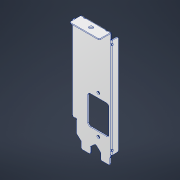
# Autodesk Inventor part: power_ac_plate
Saved by Autodesk Inventor 2022 (Build 260153000, 153)
## iProperties
Created: 2025-03-03
Part Number: power_ac_plate
Material: アルミニウム 6061
Document SubType Name: Sheet Metal
Designer: gisen
Density: 2.7 g/cm^3
Sheet Metal Rule: Default_mm
Appearance: アルミニウム - フラット
Author: gisen
Autodesk Inventor part; units mm, degrees
ref_plane "YZ Plane" through (0, 0, 0) normal (1, 0, 0) x (0, 1, 0)
ref_plane "XZ Plane" through (0, 0, 0) normal (0, 1, 0) x (-1, 0, 0)
ref_plane "XY Plane" through (0, 0, 0) normal (0, 0, 1) x (1, 0, 0)
sketch "スケッチ1" plane through (0, 0, 0) normal (0, 0, 1) x (1, 0, 0)
  line L0 (0, 11.925) -> (5.45, 7)
  line L1 (5.45, 7) -> (5.45, 0)
  line L2 (5.45, 0) -> (14.95, 0)
  line L3 (14.95, 0) -> (14.95, 7)
  line L4 (14.95, 7) -> (17, 8.8525)
  line L5 (17, 8.8525) -> (17, 119.9)
  line L6 (17, 119.9) -> (0, 119.9)
  line L7 (0, 119.9) -> (0, 11.925) construction
  line L8 (0, 11.925) -> (-5.45, 7)
  line L9 (-5.45, 7) -> (-5.45, 0)
  line L10 (-5.45, 0) -> (-14.95, 0)
  line L11 (-14.95, 0) -> (-14.95, 7)
  line L12 (-14.95, 7) -> (-17, 8.8525)
  line L13 (-17, 8.8525) -> (-17, 119.9)
  line L14 (-17, 119.9) -> (0, 119.9)
  point P0 (0, 0)
  dimension "d0" = 9.5
  dimension "d2" = 11.925
  dimension "d3" = 7
  dimension "d4" = 119.9
  dimension "d73" = 132.103
  dimension "d74" = 132.103
  dimension "d75" = 34
  measures "d0" distance of L1.end L2.end
  measures "d2" distance from line of L2 L0.start
  measures "d3" distance of L0.end L1.end
  measures "d4" distance between parallel lines of L2 L6
  measures "d73" angle of L1 L0
  measures "d74" angle of L3 L4
  measures "d75" distance between parallel lines of L5 L13
extrude "プレート1" add sketch "スケッチ1" along normal blind 1
sketch "スケッチ3" plane through (0, 0, 1) normal (0, 0, 1) x (1, 0, 0)
  line L0 (-17, 119.9) -> (17, 119.9) construction
  line L1 (-17, 8.8525) -> (-17, 119.9) construction
  line L2 (17, 119.9) -> (17, 8.8525) construction
  line L3 (0, 11.925) -> (0, 119.9) construction
  line L4 (-17, 64.3763) -> (17, 64.3763) construction
  line L5 (-8.05, 55.125) -> (14.05, 55.125)
  line L6 (14.05, 55.125) -> (14.05, 24.725)
  line L7 (14.05, 24.725) -> (-8.05, 24.725)
  line L8 (-8.05, 24.725) -> (-8.05, 55.125)
  line L9 (3, 59.925) -> (3, 19.925) construction
  circle A0 centre (3, 59.925) radius 1.55
  circle A1 centre (3, 19.925) radius 1.55
  point P0 (0, 0)
  point P1 (-8.05, 39.925)
  point P2 (3, 39.925)
  point P3 (3, 55.125)
  dimension "d77" = 22.1
  dimension "d78" = 30.4
  dimension "d79" = 40
  dimension "d80" = 3.1
  dimension "d83" = 3
  dimension "d84" = 8
  constraints: 14 end point, 6 midpoint, 2 centre point, 2 coincident, 2 parallel, 1 equal radius, 1 horizontal, 1 horizontal alignment, 1 perpendicular, 1 point on line, 1 vertical
  measures "d77" distance of L6.end L7.end
  measures "d78" distance of L5.end L6.end
  measures "d79" distance of L9.start L9.end
  measures "d80" diameter of A0
  measures "d83" distance between parallel lines of L9 L3
  measures "d84" vertical distance of L9.end L3.start
extrude "切り取り1" cut sketch "スケッチ3" against normal blind 1
sketch "スケッチ4" plane through (0, 0, 1) normal (0, 0, 1) x (1, 0, 0)
  line L0 (17, 119.9) -> (15.5, 119.9)
  line L1 (15.5, 119.9) -> (15.5, 114.3)
  line L2 (15.5, 114.3) -> (17, 114.3)
  line L3 (17, 114.3) -> (17, 119.9)
  line L4 (14.95, 7) -> (14.95, 0) construction
  line L5 (-17, 119.9) -> (-15.5, 119.9)
  line L6 (-15.5, 119.9) -> (-15.5, 114.3)
  line L7 (-15.5, 114.3) -> (-17, 114.3)
  line L8 (-17, 114.3) -> (-17, 119.9)
  point P0 (0, 0)
  dimension "d14" = 5.6
  dimension "d76" = 1.5
  constraints: 16 end point, 4 parallel, 2 equal length, 2 horizontal, 2 perpendicular
  measures "d14" distance of L0.end L1.end
  measures "d76" distance of L1.end L2.end
extrude "切り取り2" cut sketch "スケッチ4" against normal blind 1
sketch "スケッチ5" plane through (0, 0, 1) normal (0, 0, 1) x (1, 0, 0)
  line L0 (17, 8.8525) -> (14.95, 7) construction
  line L1 (17, 114.3) -> (17, 8.8525) construction
  line L2 (15.5, 7.497) -> (15.5, 10)
  line L3 (15.5, 10) -> (17, 10)
  line L4 (15.5, 7.497) -> (17, 8.8525)
  line L5 (17, 8.8525) -> (17, 10)
  line L6 (14.95, 7) -> (14.95, 0) projected
  line L7 (14.95, 0) -> (5.45, 0) projected
  line L8 (0, 11.925) -> (0, 120.3299) construction
  line L9 (-17, 8.8525) -> (-14.95, 7) construction
  line L10 (-15.5, 7.497) -> (-15.5, 10)
  line L11 (-15.5, 10) -> (-17, 10)
  line L12 (-15.5, 7.497) -> (-17, 8.8525)
  line L13 (-17, 8.8525) -> (-17, 10)
  line L14 (15.5, 114.3) -> (15.5, 119.9) construction
  point P0 (0, 0)
  dimension "d18" = 10
  constraints: 20 end point, 5 symmetric about line, 4 point on line, 2 vertical, 1 perpendicular
  measures "d18" distance between parallel lines of L7 L3
extrude "切り取り3" cut sketch "スケッチ5" against normal blind 1 contours L2 L3 L5 L4
sketch "スケッチ7" plane through (-15.5, 119.901, 1.001) normal (0, 1, 0) x (-1, 0, 0)
  line L0 (-31, 0) -> (0, 0)
  line L1 (0, 0) -> (0, 11.599)
  line L2 (0, 11.599) -> (-31, 11.599)
  line L3 (-31, 11.599) -> (-31, 0)
  constraints: 6 end point, 1 horizontal, 1 perpendicular, 1 vertical
edge flange "フランジ1" height 11.6 angle 90 thickness 1 bend radius 0 thickness toward (0, 1, 0) relief straight relief width 1 relief depth 0.5 edges at (0, 119.9, 1) wall of the first edge with corners at (15.5, 119.901, 1.001) (-15.5, 119.901, 1.001) (-15.5, 119.901, 12.6) (15.5, 119.901, 12.6)
bend "曲げ2"
corner "コーナー1"
sketch "スケッチ8" plane through (16, 10, 1) normal (1, 0, 0) x (0, 1, 0)
  line L0 (104.3, 0) -> (0, 0)
  line L1 (0, 0) -> (0, -7)
  line L2 (0, -7) -> (104.3, -7)
  line L3 (104.3, -7) -> (104.3, 0)
  constraints: 6 end point, 1 horizontal, 1 perpendicular, 1 vertical
edge flange "フランジ2" height 6 angle 90 thickness 1 bend radius 0 thickness toward (1, 0, 0) relief straight relief width 1 relief depth 0.5 edges at (17, 62.15, 0) wall of the first edge with corners at (16, 114.3, 1) (16, 10, 1) (16, 10, -6) (16, 114.3, -6)
bend "曲げ3"
corner "コーナー2"
sketch "スケッチ15" plane through (0, 0, 1) normal (0, 0, 1) x (1, 0, 0)
  line L0 (-17, 8.8525) -> (-17, 114.3)
  line L1 (-14.95, 7) -> (-17, 8.8525) construction
  line L2 (-17, 8.8525) -> (-24, 15.1782)
  line L3 (-24, 15.1782) -> (-24, 114.3)
  line L4 (-24, 114.3) -> (-17, 114.3)
  line L5 (-24, 25) -> (-20, 25)
  line L6 (-20, 25) -> (-20, 11.5635)
  line L7 (-5.45, 0) -> (-14.95, 0)
  point P0 (0, 0)
  dimension "d98" = 7
  dimension "d105" = 4
  dimension "d106" = 25
  measures "d98" distance of L3.end L0.end
  measures "d105" distance of L5.start L5.end
  measures "d106" distance between parallel lines of L7 L5
sheet face with bend "面4" sketch "スケッチ15" thickness 1 toward (0, 0, -1) bend radius 0 relief straight relief width 1 relief depth 0.5 contours L2 L6 L5 L3 L4 L0
bend "曲げ6"
sketch "スケッチ16" plane through (0, 0, 1) normal (0, 0, 1) x (1, 0, 0)
  line L0 (-24, 25) -> (-20, 25) construction
  line L1 (-20, 25) -> (-20, 11.5635) construction
  line L2 (-20, 25) -> (-20.7425, 24.2575) construction
  line L3 (-20, 25) -> (-18.95, 25) construction
  circle A0 centre (-20.7425, 24.2575) radius 1.05
  point P0 (0, 0)
  dimension "d108" = 2.1
  dimension "d107" = 135
  constraints: 4 end point, 1 coincident, 1 equal length, 1 horizontal, 3 other
  measures "d107" angle of L2 L3
extrude "切り取り7" cut sketch "スケッチ16" against normal blind 1
fillet "フィレット1" radius 1.2 6 edges at (5.45, 0, 0.5) (0, 11.925, 0.5) (14.95, 0, 0.5) (-14.95, 0, 0.5) (-5.45, 0, 0.5) (15.5, 7.497, 0.5)
fillet "フィレット2" radius 0.75 4 edges at (5.45, 7, 0.5) (14.95, 7, 0.5) (-5.45, 7, 0.5) (-14.95, 7, 0.5)
fillet "フィレット3" radius 1.2 6 edges at (16.5, 10, -6) (16.5, 114.3, -6) (-15.5, 120.401, 12.6) (15.5, 120.401, 12.6) (-24, 25, 0.5) (-24, 114.3, 0.5)
fillet "フィレット3" radius 0.5 2 edges at (-20, 23.5151, 0.5) (-21.4849, 25, 0.5)
sketch "スケッチ12" plane through (-15.5, 120.901, 1.001) normal (0, 1, 0) x (1, 0, 0)
  line L0 (15.5, 1.001) -> (15.5, -11.599) construction
  line L1 (29.8, -11.599) -> (1.2, -11.599) construction
  circle A0 centre (16.2, -5.299) radius 2
  line L2 (16.2, -5.299) -> (-4.2, -5.299)
  circle A1 centre (-4.2, -5.299) radius 2
  dimension "d68" = 6.3
  dimension "d69" = 4
  dimension "d70" = 20.4
  dimension "d104" = 0.7
  constraints: 4 end point, 2 centre point, 1 coincident, 1 equal radius, 1 horizontal, 1 midpoint, 1 vertical
  measures "d68" distance from line of L2.start L1
  measures "d69" diameter of A0
  measures "d70" distance of L2.start L2.end
  measures "d104" distance from line of L2.start L0
extrude "切り取り5" cut sketch "スケッチ12" against normal blind 1
fillet "フィレット4" radius 2.5 4 edges at (-8.05, 24.725, 0.5) (-8.05, 55.125, 0.5) (14.05, 55.125, 0.5) (14.05, 24.725, 0.5)
unfold all bends "展開1" k factor 0.44 fixed face at (0.9377, 96.6879, 1)
sketch "スケッチ13" plane through (0, 0, 1) normal (0, 0, 1) x (1, 0, 0)
  line L0 (-15.5, 120.5927) -> (-15.5, 119.9) construction
  line L1 (15.5, 120.5927) -> (15.5, 119.9) construction
  line L2 (15.999, 114.3) -> (16.6917, 114.3) construction
  line L3 (16.6917, 10) -> (15.999, 10) construction
  circle A0 centre (-11.5, 120.2464) radius 1.05
  circle A1 centre (11.5, 120.2464) radius 1.05
  circle A2 centre (16.3454, 110.3) radius 1.05
  circle A3 centre (16.3454, 14) radius 1.05
  point P0 (0, 0)
  point P1 (-15.5, 120.2464)
  point P2 (16.3454, 114.3)
  dimension "d85" = 2.1
  dimension "d86" = 4
  dimension "d87" = 4
  dimension "d88" = 4
  dimension "d89" = 4
  constraints: 4 centre point, 3 equal radius, 2 horizontal alignment, 2 midpoint, 2 vertical alignment
  measures "d85" diameter of A0
  measures "d86" distance of A0.centre point (-15.5, 120.246)
  measures "d87" distance from line of L1 A1.centre
  measures "d88" distance of A2.centre point (16.345, 114.3)
  measures "d89" distance from line of L3 A3.centre
extrude "切り取り6" cut sketch "スケッチ13" against normal blind 1
refold all bends "再折り曲げ1"
equation "\"d88\" = d87"
equation "\"d74\" = d73"
equation "\"d11\" = Thickness"
equation "\"d15\" = Thickness"
equation "\"d19\" = Thickness"
equation "\"d109\" = Thickness"
equation "\"d71\" = Thickness"
equation "\"d87\" = d86"
equation "\"d89\" = d88"
equation "\"d90\" = Thickness"
equation "\"d5\" = Thickness"
equation "\"d33\" = BendReliefWidth"
equation "\"d34\" = BendReliefDepth"
equation "\"d35\" = MinimumRemnant"
equation "\"d40\" = CornerReliefSize"
equation "\"d41\" = GapSize"
equation "\"d43\" = BendReliefWidth"
equation "\"d44\" = BendReliefDepth"
equation "\"d45\" = MinimumRemnant"
equation "\"d50\" = CornerReliefSize"
equation "\"d51\" = GapSize"
equation "\"d100\" = BendReliefWidth"
equation "\"d102\" = MinimumRemnant"
equation "\"d101\" = BendReliefDepth"
equation "\"BendReliefWidth\" = Thickness"
equation "\"BendReliefDepth\" = 0.5 * Thickness"
equation "\"CornerReliefSize\" = 4 * Thickness"
equation "\"MinimumRemnant\" = 2 * Thickness"
equation "\"GapSize\" = Thickness"
equation "\"Thickness\" = 1"
